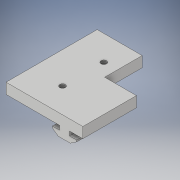
# Autodesk Inventor part: Sliderfor2020
Saved by Autodesk Inventor 2017 (Build 210142000, 142)
## iProperties
Created: 2017-12-08
Part Number: Sliderfor2020
Material: Generic
Document SubType Name: Modeling
Designer: User
Density: 1 g/cm^3
Appearance: Default
Author: User
Autodesk Inventor part; units mm, degrees
ref_plane "YZ Plane" through (0, 0, 0) normal (1, 0, 0) x (0, 1, 0)
ref_plane "XZ Plane" through (0, 0, 0) normal (0, 1, 0) x (-1, 0, 0)
ref_plane "XY Plane" through (0, 0, 0) normal (0, 0, 1) x (1, 0, 0)
sketch "Sketch1" plane through (0, 0, 0) normal (0, 0, 1) x (1, 0, 0)
  line L0 (0, 0) -> (14.5304, 0)
  line L1 (-8.7854, 6.6412) -> (8.5466, 6.6412)
  line L2 (8.5466, 1.6412) -> (2.2606, 1.6412)
  line L3 (2.2606, 1.6412) -> (2.2606, -0.3588)
  line L4 (2.2606, -0.3588) -> (5.6256, -0.3588)
  line L5 (2.5721, -3.1588) -> (-3.1429, -3.1588)
  line L6 (-3.1429, -3.1588) -> (-5.8644, -1.1208)
  line L7 (-5.8644, -1.1208) -> (-5.8644, -0.3588)
  line L8 (-5.8644, -0.3588) -> (-2.4994, -0.3588)
  line L9 (-2.4994, -0.3588) -> (-2.4994, 1.6412)
  line L10 (-2.4994, 1.6412) -> (-8.7854, 1.6412)
  line L11 (-8.7854, 1.6412) -> (-8.7854, 6.6412)
  line L12 (5.6256, -0.3588) -> (5.6256, -1.1208)
  line L13 (5.6256, -1.1208) -> (2.5721, -3.1588)
  line L14 (8.5466, 6.6412) -> (5.0156, 6.6412)
  line L15 (5.0156, 1.6412) -> (8.5466, 1.6412)
  line L16 (8.5466, 6.6412) -> (8.5466, 1.6412)
  dimension "d2" = 5
  dimension "d3" = 2
  dimension "d6" = 11.49
  dimension "d7" = 2.921
  dimension "d9" = 5.6425
  dimension "d11" = 0.762
  dimension "d12" = 0.762
  dimension "d78" = 2.921
  dimension "d88" = 3.365
  dimension "d89" = 3.365
  constraints: 34 end point, 5 perpendicular, 4 point on line, 3 horizontal, 2 vertical, 1 collinear
  measures "d2" distance between parallel lines of L10 L1
  measures "d3" distance between parallel lines of L8 L10
  measures "d6" distance between parallel lines of L7 L12
  measures "d7" distance between parallel lines of L7 L11
  measures "d9" distance from line of L5.end L11
  measures "d11" distance of L6.end L7.end
  measures "d12" distance of L4.end L12.end
  measures "d78" distance between parallel lines of L16 L12
  measures "d88" distance between parallel lines of L9 L7
  measures "d89" distance from line of L4.end L3
extrude "Extrusion1" add sketch "Sketch1" along normal blind 25.4
sketch "Sketch7" plane through (-8.7854, 1.6412, 0) normal (-1, 0, 0) x (0, 0, 1)
  line L0 (0, 0) -> (0, 5) projected
  line L1 (0, 0) -> (25.4, 0) projected
  line L2 (25.4, 5) -> (25.4, 0) projected
  line L3 (0, 5) -> (25.4, 5) projected
  point P0 (0, -1.6412)
extrude "Extrusion4" add sketch "Sketch7" along normal blind 25.4
thicken "Thicken1" operation add thickness 6.35 both sides no extend neighbours yes toward (1, 0, 0) faces at (-34.1854, 4.9745, 8.4667)
sketch "Sketch10" plane through (0, 0, 0) normal (0, 0, -1) x (-1, 0, 0)
  line L0 (-8.5466, 6.6412) -> (27.8354, 6.6412) projected
  line L1 (2.4994, 1.6412) -> (27.8354, 1.6412) projected
  line L2 (27.8354, 6.6412) -> (6.5139, 6.6412)
  line L3 (6.5139, 6.6412) -> (6.5139, 1.6412)
  line L4 (6.5139, 1.6412) -> (27.8354, 1.6412)
  line L5 (27.8354, 1.6412) -> (27.8354, 6.6412)
  point P0 (0, 0)
  constraints: 8 end point, 2 parallel, 1 horizontal, 1 perpendicular, 1 point on line
extrude "Extrusion5" add sketch "Sketch10" along normal blind 17.78
sketch "Sketch13" plane through (8.5466, 6.6412, 25.4) normal (0, 1, 0) x (1, 0, 0)
  line L0 (-36.382, 0) -> (-36.382, 43.18) projected
  line L1 (0, 0) -> (-36.382, 0) projected
  line L2 (0, 25.4) -> (0, 0) projected
  line L3 (-15.0605, 25.4) -> (0, 25.4) projected
  line L4 (-15.0605, 25.4) -> (-15.0605, 43.18) projected
  line L5 (-36.382, 43.18) -> (-15.0605, 43.18) projected
  point P0 (-8.5466, 25.4)
  point P1 (-21.4105, 31.369)
  point P2 (-21.4105, 11.811)
  dimension "d149" = 43.18
  dimension "d150" = 19.558
  dimension "d151" = 11.811
  dimension "d152" = 6.35
  dimension "d153" = 6.35
  measures "d149" distance between parallel lines of L1 L5
  measures "d150" distance of point (-21.411, 11.811) point (-21.411, 31.369)
  measures "d151" distance from line of L5 point (-21.411, 31.369)
  measures "d152" distance from line of L4 point (-21.411, 31.369)
  measures "d153" distance from line of L4 point (-21.411, 11.811)
hole "Hole8" at (-12.8639, 6.6412, -5.969) at (-12.8639, 6.6412, 13.589) direction (0, -1, 0) diameter 2.6416 depth 10.9728 tip angle 118 thread size "6-32 UNC" class "2B" standard "ANSI Unified Screw Threads"
equation "\"d9\" = -0.5 * d8 + 0.5 * d0"
equation "\"d12\" = d11"
equation "\"d151\" = -0.5 * d150 + 0.5 * d149"
equation "\"d8\" = 5.715"
equation "\"d0\" = 17"
body "Solid1"
